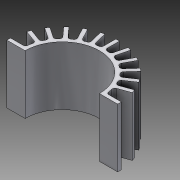
# Autodesk Inventor part: HEAT SINK, CIM MOTOR AndyMark FR801-001
Saved by Autodesk Inventor 2015 (Build 190159000, 159)
## iProperties
Created: 2015-01-15
Part Number: HEAT SINK, CIM MOTOR AndyMark FR801-001
Material: Aluminum 6061
Document SubType Name: Modeling
Designer: TODD D MILLER
Mass: 120.753 g
Surface Area: 286.534 cm^2
Volume: 44.7232 cm^3
Density: 2.7 g/cm^3
Appearance: Aluminum - Flat
Author: TODD D MILLER
Autodesk Inventor part; units mm, degrees
note: some values were not read from the file. Chosen so that the rebuilt part matches the saved one: pattern direction of "Circular Pattern1".
ref_plane "YZ Plane" through (0, 0, 0) normal (1, 0, 0) x (0, 1, 0)
ref_plane "XZ Plane" through (0, 0, 0) normal (0, 1, 0) x (-1, 0, 0)
ref_plane "XY Plane" through (0, 0, 0) normal (0, 0, 1) x (1, 0, 0)
sketch "Sketch1" plane through (0, 0, 0) normal (0, 1, 0) x (-1, 0, 0)
  arc A0 (-32.131, 0) -> (32.131, 0) centre (0, 0) ccw
  circle A1 centre (0, 0) radius 48.006 construction
  arc A2 (-35.306, 0) -> (35.306, 0) centre (0, 0) ccw
  arc A3 (35.306, 0) -> (-35.306, 0) centre (0, 0) ccw construction
  arc A4 (32.131, 0) -> (-32.131, 0) centre (0, 0) ccw construction
  line L0 (-32.131, 0) -> (-35.306, 0)
  line L1 (1.5875, -47.9797) -> (-1.5875, -47.9797)
  line L2 (-1.5875, -47.9797) -> (-1.5875, -32.131)
  line L3 (-1.5875, -32.131) -> (1.5875, -32.131)
  line L4 (1.5875, -32.131) -> (1.5875, -47.9797)
  line L5 (-67.2084, 0) -> (67.2084, 0) construction
  line L6 (35.306, 0) -> (32.131, 0)
  line L7 (32.131, 0) -> (47.9009, 0)
  line L8 (47.9009, 0) -> (47.9009, -3.175)
  line L9 (47.9009, -3.175) -> (32.131, -3.175)
  line L10 (32.131, -3.175) -> (32.131, 0)
  point P0 (0, -32.131)
  dimension "d0" = 64.262
  dimension "d1" = 15.875
  dimension "d2" = 3.175
  dimension "d3" = 3.175
  dimension "d5" = 3.175
  constraints: 20 end point, 11 point on circle, 5 centre point, 4 parallel, 3 horizontal, 2 perpendicular, 1 coincident, 1 collinear, 1 midpoint, 1 point on line
  measures "d0" diameter of A0
  measures "d1" radial gap between concentric circles of A1 A0
  measures "d2" radial gap between concentric circles of A0 A2
  measures "d3" distance of L1.start L1.end
  measures "d5" distance of L7.end L8.end
extrude "Extrusion1" add sketch "Sketch1" along normal mid plane 50.8 contours A0 L3 L2 A2 L0 | L3 L4 A2 L2 | A0 L10 L9 A2 L4 L3 | L6 A2 L9 L10
extrude "Extrusion2" add sketch "Sketch1" against normal up to surface (50.8 mm away) from surface at 25.4 contours L3 L4 A2 L2 | A2 L4 L1 L2
pattern_circular "Circular Pattern1" count 11 over 140 about axis through (0, -10, 0) along (0, 1, 0) of "Extrusion2" both ways yes
extrude "Extrusion3" add sketch "Sketch1" against normal up to surface (50.8 mm away) from surface at 25.4 contours L6 A2 L9 L10 | L7 L8 L9 A2
mirror "Mirror1" about plane through (0, 0, 0) normal (1, 0, 0) of "Extrusion3"
fillet "Fillet1" radius 2.2225 24 edges at (-35.1629, 0, -3.175) (-30.1281, 0, -18.4068) (-17.9601, 0, -30.3965) (-32.6003, 0, -13.5549) (-33.6862, 0, -10.5714) (-22.4207, 0, -27.2732) (-24.7802, 0, -25.1487) (-6.9923, 0, -34.6067) (-10.073, 0, -33.8386) (17.9601, 0, -30.3965) (15.1567, 0, -31.8871) (30.1281, 0, -18.4068) (28.3527, 0, -21.039) (1.5875, 0, -35.2703) (-1.5875, 0, -35.2703) (-15.1567, 0, -31.8871) (6.9923, 0, -34.6067) (22.4207, 0, -27.2732) (32.6003, 0, -13.5549) (24.7802, 0, -25.1487) (10.073, 0, -33.8386) (35.1629, 0, -3.175) (33.6862, 0, -10.5714) (-28.3527, 0, -21.039)
equation "\"d3\" = d2"
equation "\"d5\" = d2"
body "Solid1"
